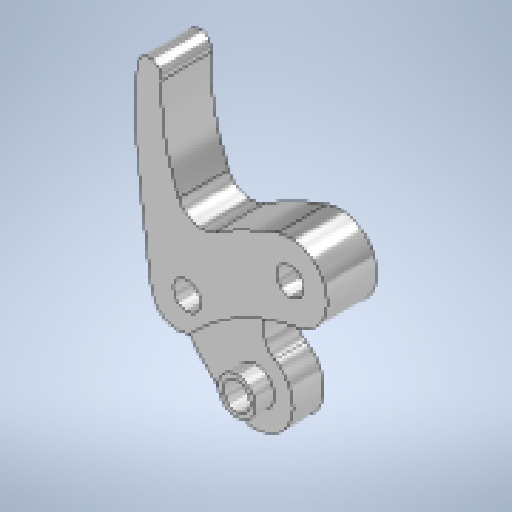
# Autodesk Inventor part: Lever
Saved by Autodesk Inventor 2023.2 (Build 272271000, 271)
## iProperties
Created: 2024-01-16
Part Number: Lever
Material: Aluminum 6061
Document SubType Name: Modeling
Designer: Nathan Cai
Mass: 6.36377 g
Surface Area: 16.7426 cm^2
Volume: 2.35695 cm^3
Density: 2.7 g/cm^3
Appearance: Aluminum - Flat
Pivot_x: 0.594 in
Pivot_y: 0.125 in
Angle_Offset: 20.00 deg
Author: Nathan Cai
Autodesk Inventor part; units mm, degrees
ref_plane "YZ Plane" through (0, 0, 0) normal (1, 0, 0) x (0, 1, 0)
ref_plane "XZ Plane" through (0, 0, 0) normal (0, 1, 0) x (-1, 0, 0)
ref_plane "XY Plane" through (0, 0, 0) normal (0, 0, 1) x (1, 0, 0)
sketch "Sketch1" plane through (0, 0, 0) normal (0, 0, 1) x (1, 0, 0)
  circle A0 centre (0, 0) radius 1.7526
  circle A1 centre (0, 0) radius 4.7625
  circle A2 centre (0, 0) radius 19.05 construction
  circle A3 centre (0, 19.05) radius 3.175 construction
  line L0 (0, 19.05) -> (0, 0) construction
  line L1 (0, 19.05) -> (3.175, 19.05) construction
  arc A4 (-3.1628, 22.1199) -> (-6.3202, 22.4358) centre (-4.7468, 22.225) ccw
  arc A5 (-6.3202, 22.4358) -> (-6.3695, 12.7) centre (31.4424, 17.3766) ccw
  line L2 (-6.3695, 12.7) -> (-4.7265, -0.5846)
  circle A6 centre (13.0858, 8.1416) radius 6.35 construction
  line L3 (7.1188, 5.9698) -> (13.0858, 8.1416) construction
  line L4 (0, 0) -> (-3.1615, 8.6862) construction
  circle A7 centre (13.0858, 8.1416) radius 1.7526
  circle A8 centre (13.0858, 8.1416) radius 4.7625
  arc A9 (-3.1628, 22.1199) -> (3.5023, 3.2272) centre (22.1815, 20.4391) ccw
  arc A10 (11.457, 12.6169) -> (-3.295, 3.4387) centre (25.8792, -27.008) ccw
  line L5 (11.457, 12.6169) -> (7.5101, 11.1804) construction
  arc A11 (13.9098, 3.4509) -> (3.8438, -2.8118) centre (16.6566, -12.1846) ccw
  circle A12 centre (6.35, -7.9375) radius 6.35 construction
  circle A13 centre (6.35, -7.9375) radius 1.7526
  circle A14 centre (6.35, -7.9375) radius 4.7625
  arc A15 (14.3671, 3.5547) -> (10.518, -5.6334) centre (16.0754, -2.5612) ccw
  arc A16 (-4.534, -1.4576) -> (3.9327, -12.0409) centre (13.6019, 4.3728) ccw
  arc A17 (8.88, 5.9072) -> (4.9925, -3.3726) centre (16.0754, -2.5612) ccw
  arc A18 (2.1929, -4.2276) -> (2.7069, -4.8701) centre (13.6019, 4.3728) ccw
  arc A19 (8.7233, 6.2311) -> (3.6415, 3.0694) centre (25.8792, -27.008) ccw
  circle A20 centre (0, 0) radius 3.175 construction
  point P0 (3.7177, 2.9766)
  point P1 (0.7293, 6.839)
  point P2 (4.2726, -2.1039)
  point P3 (-4.7377, -0.494)
  point P4 (1.4187, -4.5463)
  point P5 (3.3438, -3.3912)
  point P6 (5.0258, -1.3799)
  dimension "d1" = 9.525
  dimension "d2" = 38.1
  dimension "d3" = 6.35
  dimension "d0" = 3.5052
  dimension "d5" = 3.175
  dimension "d6" = 3.175
  dimension "d7" = 38.1
  dimension "d8" = 6.35
  dimension "d11" = 12.7
  dimension "d12" = 3.5052
  dimension "Pivot_x" = 15.0813
  dimension "Pivot_y" = 3.175
  dimension "d16" = 9.525
  dimension "d18" = 25.4
  dimension "d19" = 15.875
  dimension "d21" = 12.7
  dimension "d22" = 3.5052
  dimension "d23" = 7.9375
  dimension "d24" = 6.35
  dimension "d25" = 9.525
  dimension "d26" = 6.35
  dimension "d27" = 4.7625
  dimension "d28" = 4.7625
  dimension "d29" = 4.7625
  dimension "d31" = 19.05
  dimension "Angle_Offset" = 20
  dimension "d33" = 6.35
  constraints: 32 point on circle, 18 centre point, 12 end point, 10 tangent, 8 coincident, 1 horizontal, 1 horizontal alignment, 1 parallel, 1 perpendicular, 1 vertical, 1 vertical alignment, 20 other
  measures "d0" diameter of A0
  measures "d5" diameter of A4
  measures "d6" distance from line of L1 A4.centre
  measures "d7" radius of A5
  measures "d8" distance from line of L1 L2.start
  measures "d11" diameter of A6
  measures "d12" diameter of A7
  measures "Pivot_x" distance from line of L4 L3.end
  measures "Pivot_y" distance from line of point (0, 0) L3
  measures "d16" diameter of A8
  measures "d18" radius of A9
  measures "d19" radius of A11
  measures "d21" diameter of A12
  measures "d22" diameter of A13
  measures "d23" vertical distance of A13.centre point (0, 0)
  measures "d24" horizontal distance of A0.centre A13.centre
  measures "d25" diameter of A14
  measures "d26" radius of A15
  measures "d27" radial gap between concentric circles of A15 A17
  measures "d28" radial gap between concentric circles of A16 A18
  measures "d29" radial gap between concentric circles of A10 A19
  measures "d31" radius of A16
  measures "Angle_Offset" angle of L0 L4
  measures "d33" diameter of A20
extrude "Extrusion1" add sketch "Sketch1" along normal blind 6.35 contours A1 | A1 A19 A8 A17 A11 | A1 A9 A10 A8 A19 | A11 A17 A14 A18 A1 | A1 A10 A9 | A8 | A18 A14 A16 A1 | A17 A8 A11 | A1 L2 A5 A4 A9 A10 | A14
fillet "Fillet1" radius 3.175 1 edges at (0.7293, 6.839, 3.175)
fillet "Fillet2" [suppressed]
fillet "Fillet3" radius 3.175 2 edges at (5.0258, -1.3799, 3.175) (4.9925, -3.3726, 3.175)
chamfer "Chamfer1" distance 2.3813 angle 45 1 edges at (4.5974, -7.9375, 0)
sketch "Sketch3" plane through (0, 0, 6.35) normal (0, 0, 1) x (1, 0, 0)
  circle A0 centre (6.35, -7.9375) radius 1.7526 projected
  circle A1 centre (6.35, -7.9375) radius 6.9538
  arc A2 (13.9098, 3.4509) -> (11.457, 12.6169) centre (13.0858, 8.1416) ccw projected
  arc A3 (13.9098, 3.4509) -> (1.4494, -3.004) centre (17.9645, -19.6301) ccw
  arc A4 (13.9098, 3.4509) -> (8.8593, 1.6435) centre (16.6566, -12.1846) ccw projected
  line L0 (13.9098, 3.4509) -> (13.2943, -8.3012)
  circle A5 centre (0, 0) radius 3.175
  circle A6 centre (6.35, -7.9375) radius 2.3813
  dimension "d42" = 6.35
  dimension "d43" = 4.7625
  constraints: 4 centre point, 4 point on circle, 4 tangent, 3 coincident, 2 end point
  measures "d42" diameter of A5
  measures "d43" diameter of A6
extrude "Extrusion2" cut sketch "Sketch3" against normal blind 2.3813 contours A1 | A1 A3 L0
fillet "Fillet4" radius 3.175 1 edges at (-0.5926, -8.3324, 5.1594)
body "Solid1"
